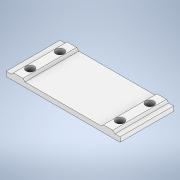
# Autodesk Inventor part: Platina
Saved by Autodesk Inventor 2022 (Build 260153000, 153)
## iProperties
Created: 2021-10-23
Part Number: Platina
Material: PET Plastic
Document SubType Name: Modeling
Designer: juanp
Density: 1.541 g/cm^3
Appearance: Polycarbonate - Clear
Author: juanp
Autodesk Inventor part; units mm, degrees
ref_plane "YZ Plane" through (0, 0, 0) normal (1, 0, 0) x (0, 1, 0)
ref_plane "XZ Plane" through (0, 0, 0) normal (0, 1, 0) x (-1, 0, 0)
ref_plane "XY Plane" through (0, 0, 0) normal (0, 0, 1) x (1, 0, 0)
sketch "Sketch1" plane through (0, 0, 0) normal (0, 1, 0) x (-1, 0, 0)
  line L0 (28.75, 9.525) -> (-28.75, 9.525) construction
  line L1 (-28.75, 9.525) -> (-28.75, -9.525) construction
  line L2 (-28.75, -9.525) -> (28.75, -9.525) construction
  line L3 (28.75, -9.525) -> (28.75, 9.525) construction
  line L4 (28.75, 9.525) -> (-28.75, -9.525) construction
  line L5 (-28.75, 9.525) -> (28.75, -9.525) construction
  circle A0 centre (28.75, 9.525) radius 2.65
  circle A1 centre (28.75, -9.525) radius 2.65
  circle A2 centre (-28.75, 9.525) radius 2.65
  circle A3 centre (-28.75, -9.525) radius 2.65
  line L6 (36.4, 17.175) -> (-36.4, 17.175)
  line L7 (-36.4, 17.175) -> (-36.4, -17.175)
  line L8 (-36.4, -17.175) -> (36.4, -17.175)
  line L9 (36.4, -17.175) -> (36.4, 17.175)
  line L10 (36.4, 17.175) -> (-36.4, -17.175) construction
  line L11 (-36.4, 17.175) -> (36.4, -17.175) construction
  point P0 (0, 0)
  dimension "d0" = 19.05
  dimension "d1" = 57.5
  dimension "d2" = 5.3
  dimension "d3" = 5
  dimension "d4" = 5
  constraints: 24 end point, 4 centre point, 4 coincident, 4 midpoint, 4 parallel, 3 equal radius, 2 horizontal, 2 perpendicular
  measures "d0" distance of L2.end L0.start
  measures "d1" distance of L1.end L2.end
  measures "d2" diameter of A1
  measures "d3" distance edge to line of A3 L7
  measures "d4" distance edge to line of A3 L8
extrude "Extrusion1" add sketch "Sketch1" along normal blind 3
sketch "Sketch2" plane through (0, 3, 0) normal (0, 1, 0) x (1, 0, 0)
  line L0 (36.4, -17.175) -> (36.4, 17.175) projected
  line L1 (36.4, 17.175) -> (-36.4, 17.175) projected
  line L2 (-36.4, 17.175) -> (-36.4, -17.175) projected
  line L3 (-36.4, -17.175) -> (36.4, -17.175) projected
  circle A0 centre (-28.75, -9.525) radius 2.65 projected
  circle A1 centre (-28.75, 9.525) radius 2.65 projected
  circle A2 centre (28.75, -9.525) radius 2.65 projected
  circle A3 centre (28.75, 9.525) radius 2.65 projected
  line L4 (-24.375, 17.175) -> (-33.125, 17.175)
  line L5 (-33.125, 17.175) -> (-33.125, -17.175)
  line L6 (-33.125, -17.175) -> (-24.375, -17.175)
  line L7 (-24.375, -17.175) -> (-24.375, 17.175)
  line L8 (-28.75, -17.175) -> (-28.75, 17.175) construction
  line L9 (33.125, 17.175) -> (24.375, 17.175)
  line L10 (24.375, 17.175) -> (24.375, -17.175)
  line L11 (24.375, -17.175) -> (33.125, -17.175)
  line L12 (33.125, -17.175) -> (33.125, 17.175)
  line L13 (28.75, 17.175) -> (28.75, -17.175) construction
  line L14 (36.4, 17.175) -> (-36.4, 17.175) projected
  line L15 (-36.4, -17.175) -> (36.4, -17.175) projected
  dimension "d14" = 8.75
  constraints: 20 end point, 5 collinear, 4 midpoint, 4 parallel, 2 horizontal, 2 perpendicular, 2 point on line
  measures "d14" distance of L4.start L4.end
extrude "Extrusion2" add sketch "Sketch2" along normal blind 1.35 contours L3 L10 L1 L12 | L3 L5 L1 L7
chamfer "Chamfer2" distance 1.35 angle 45 4 edges at (-33.125, 4.35, 0) (-24.375, 4.35, 0) (24.375, 4.35, 0) (33.125, 4.35, 0)
body "Solid1"
